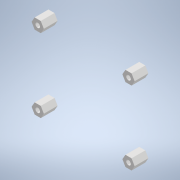
# Autodesk Inventor part: oled__stoyki
Saved by Autodesk Inventor 2022 (Build 260153000, 153)
## iProperties
Created: 2023-03-13
Part Number: oled__stoyki
Material: Типовые
Document SubType Name: Modeling
Designer: akapu
Density: 1 g/cm^3
Appearance: По умолчанию
Author: akapu
Autodesk Inventor part; units mm, degrees
ref_plane "YZ Plane" through (0, 0, 0) normal (1, 0, 0) x (0, 1, 0)
ref_plane "XZ Plane" through (0, 0, 0) normal (0, 1, 0) x (-1, 0, 0)
ref_plane "XY Plane" through (0, 0, 0) normal (0, 0, 1) x (1, 0, 0)
sketch "Эскиз1" plane through (0, 0, 0) normal (0, 0, 1) x (1, 0, 0)
  line L0 (188.3541, 393.8303) -> (208.9719, 357.8143) projected
  arc A0 (188.3541, 393.8303) -> (186.3071, 394.3869) centre (187.0523, 393.0851) ccw projected
  line L1 (179.4451, 390.4587) -> (186.3071, 394.3869) projected
  line L2 (183.1303, 384.0212) -> (179.4451, 390.4587) projected
  line L3 (182.954, 383.9203) -> (183.1303, 384.0212) projected
  line L4 (179.2688, 390.3577) -> (182.954, 383.9203) projected
  line L5 (163.8383, 381.5243) -> (179.2688, 390.3577) projected
  line L6 (167.5235, 375.0869) -> (163.8383, 381.5243) projected
  line L7 (167.3471, 374.9859) -> (167.5235, 375.0869) projected
  line L8 (163.6619, 381.4234) -> (167.3471, 374.9859) projected
  line L9 (156.7999, 377.4951) -> (163.6619, 381.4234) projected
  arc A1 (156.7999, 377.4951) -> (156.2434, 375.4481) centre (157.5452, 376.1933) ccw projected
  line L10 (157.9982, 372.3827) -> (156.2434, 375.4481) projected
  arc A2 (157.9982, 372.3827) -> (161.0468, 371.2843) centre (160.1679, 373.6247) ccw projected
  line L11 (175.7028, 345.6825) -> (161.0468, 371.2843) projected
  arc A3 (175.7028, 345.6825) -> (175.1064, 342.4975) centre (177.276, 343.7396) ccw projected
  line L12 (176.8612, 339.4321) -> (175.1064, 342.4975) projected
  arc A4 (176.8612, 339.4321) -> (178.9082, 338.8755) centre (178.163, 340.1773) ccw projected
  line L13 (208.4154, 355.7673) -> (178.9082, 338.8755) projected
  arc A5 (208.4154, 355.7673) -> (208.9719, 357.8143) centre (207.6701, 357.069) ccw projected
  circle A6 centre (178.5341, 341.542) radius 1 projected
  circle A7 centre (188.1353, 346.7502) radius 0.4445 projected
  circle A8 centre (190.3396, 348.0122) radius 0.4445 projected
  circle A9 centre (206.3055, 357.4401) radius 1 projected
  circle A10 centre (194.7483, 350.536) radius 0.4445 projected
  circle A11 centre (158.9098, 375.8223) radius 1 projected
  circle A12 centre (192.544, 349.2741) radius 0.4445 projected
  circle A13 centre (196.9527, 351.7979) radius 0.4445 projected
  circle A14 centre (199.157, 353.0598) radius 0.4445 projected
  circle A15 centre (186.6812, 391.7204) radius 1 projected
  line L14 (182.8151, 357.3203) -> (174.7893, 371.34) projected
  line L15 (182.7868, 357.2163) -> (182.8151, 357.3203) projected
  line L16 (183.8468, 355.3646) -> (182.7868, 357.2163) projected
  line L17 (180.915, 353.6863) -> (183.8468, 355.3646) projected
  line L18 (180.915, 353.6863) -> (181.4829, 352.6943) projected
  line L19 (181.4829, 352.6943) -> (179.7635, 351.71) projected
  line L20 (179.7635, 351.71) -> (178.0978, 354.6198) projected
  line L21 (178.0978, 354.6198) -> (178.6268, 354.9226) projected
  line L22 (170.6137, 368.9203) -> (178.6268, 354.9226) projected
  line L23 (170.6137, 368.9203) -> (170.0846, 368.6174) projected
  line L24 (170.0846, 368.6174) -> (168.4189, 371.5272) projected
  line L25 (168.4189, 371.5272) -> (170.1383, 372.5115) projected
  line L26 (170.1383, 372.5115) -> (170.6935, 371.5415) projected
  line L27 (173.6694, 373.2451) -> (170.6935, 371.5415) projected
  line L28 (173.6411, 373.1411) -> (173.6694, 373.2451) projected
  line L29 (174.7011, 371.2895) -> (173.6411, 373.1411) projected
  line L30 (174.7893, 371.34) -> (174.7011, 371.2895) projected
  circle A16 centre (185.9309, 345.4883) radius 0.4445 projected
  line L31 (186.6812, 391.7204) -> (186.6812, 394.0204)
  line L32 (206.3055, 357.4401) -> (204.3094, 356.2974)
  line L33 (158.9098, 375.8223) -> (158.9098, 373.5223)
  line L34 (178.5341, 341.542) -> (178.5341, 339.242)
  line L35 (157.5819, 373.5223) -> (156.254, 375.8223)
  line L36 (156.254, 375.8223) -> (157.5819, 378.1223)
  line L37 (157.5819, 378.1223) -> (160.2378, 378.1223)
  line L38 (160.2378, 378.1223) -> (161.5657, 375.8223)
  line L39 (161.5657, 375.8223) -> (160.2378, 373.5223)
  line L40 (160.2378, 373.5223) -> (157.5819, 373.5223)
  line L41 (188.0091, 394.0204) -> (189.3371, 391.7204)
  line L42 (189.3371, 391.7204) -> (188.0091, 389.4204)
  line L43 (188.0091, 389.4204) -> (185.3533, 389.4204)
  line L44 (185.3533, 389.4204) -> (184.0254, 391.7204)
  line L45 (184.0254, 391.7204) -> (185.3533, 394.0204)
  line L46 (185.3533, 394.0204) -> (188.0091, 394.0204)
  line L47 (203.6497, 357.4498) -> (204.986, 359.7449)
  line L48 (204.986, 359.7449) -> (207.6418, 359.7352)
  line L49 (207.6418, 359.7352) -> (208.9612, 357.4303)
  line L50 (208.9612, 357.4303) -> (207.6249, 355.1352)
  line L51 (207.6249, 355.1352) -> (204.9691, 355.145)
  line L52 (204.9691, 355.145) -> (203.6497, 357.4498)
  line L53 (177.2062, 339.242) -> (175.8782, 341.542)
  line L54 (175.8782, 341.542) -> (177.2062, 343.842)
  line L55 (177.2062, 343.842) -> (179.862, 343.842)
  line L56 (179.862, 343.842) -> (181.1899, 341.542)
  line L57 (181.1899, 341.542) -> (179.862, 339.242)
  line L58 (179.862, 339.242) -> (177.2062, 339.242)
  point P0 (0, 0)
  dimension "d0" = 2.3
  dimension "d1" = 2.3
  dimension "d2" = 2.3
  dimension "d3" = 2.3
  constraints: 56 end point, 4 coincident, 4 midpoint, 3 vertical, 1 parallel, 52 other
  measures "d0" distance of L31.start L31.end
  measures "d1" distance of L33.start L33.end
  measures "d2" distance of L34.start L34.end
  measures "d3" distance of L32.start L32.end
extrude "Выдавливание1" add sketch "Эскиз1" along normal blind 6 contours L46 L41 L42 L43 L44 L45 L1 | L1 L45 L46 | L50 L51 L13 | L13 L51 L52 L47 L48 L49 L50 | L57 L58 L13 | L13 L58 L53 L54 L55 L56 L57 | L37 L38 L39 L40 L35 L36 L9 | L9 L36 L37
